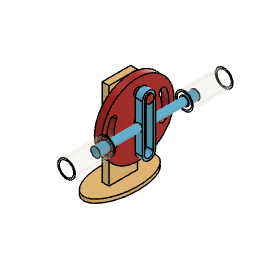
Scotch Yoke Mechanism v7 (Autodesk Fusion 360 design; units mm, degrees)
Autodesk Fusion 360 part; units mm, degrees
sketch "crank and pin" plane through (0, 0, 0) normal (1, 0, 0) x (0, 1, 0) in component "crank"
  circle A0 centre (0, 0) radius 50
  circle A1 centre (0, 33) radius 6
  line L0 (-50, 0) -> (50, 0) construction
  line L1 (0, 50) -> (0, -50) construction
  arc A2 (-30.2565, 13.1735) -> (-39.3225, 17.3995) centre (-34.4333, 16.0506) ccw
  arc A3 (-39.3225, -17.3995) -> (-30.2565, -13.1735) centre (-34.4333, -16.0506) ccw
  arc A4 (-38.6101, 18.9278) -> (-38.6101, -18.9278) centre (0, 0) ccw
  arc A5 (-29.5442, 14.7018) -> (-29.5442, -14.7018) centre (0, 0) ccw
  arc A6 (29.5442, -14.7018) -> (29.5442, 14.7018) centre (0, 0) ccw
  arc A7 (38.6101, -18.9278) -> (38.6101, 18.9278) centre (0, 0) ccw
  arc A8 (39.3225, 17.3995) -> (30.2565, 13.1735) centre (34.4333, 16.0506) ccw
  arc A9 (30.2565, -13.1735) -> (39.3225, -17.3995) centre (34.4333, -16.0506) ccw
  circle A10 centre (0, 0) radius 5
  dimension "d1" = 100
  dimension "d2" = 12
  dimension "d27" = 10
  constraint coincident A0.centre A4.centre
  constraint coincident A0 L0.start
  constraint coincident A0 L0.end
  constraint horizontal L0
  constraint coincident A0 L1.start
  constraint coincident A0 L1.end
  constraint vertical L1
  constraint symmetric L0 A2 A3
  constraint coincident A3 A4.end
  constraint coincident A3 A5.end
  constraint coincident A2 A4.start
  constraint coincident A2 A5.start
  constraint symmetric L1 A2.end A8.start
  constraint symmetric L1 A2.start A8.end
  constraint symmetric L1 A2 A8
  constraint symmetric L1 A3.end A9.start
  constraint symmetric L1 A3.start A9.end
  constraint symmetric L1 A3 A9
  constraint symmetric L1 A4.end A7.start
  constraint symmetric L1 A5.end A6.start
  constraint symmetric L1 A4.start A7.end
  constraint symmetric L1 A4 A7
  constraint symmetric L1 A5.start A6.end
  constraint symmetric L1 A5 A6
  constraint concentric A0 A10
  measures "d1" diameter of A0
  measures "d2" diameter of A1
  measures "d27" diameter of A10
extrude "Extrude1" add sketch "crank and pin" along normal blind 10 contours A0 | A1 | A2 A5 | A2 A3 A4 A5 | A3 A5 | A2 A4 | A3 A4 | A6 A9 | A6 A7 A8 A9 | A7 A9 | A6 A8 | A7 A8 | A10 makes body 1 in component "crank"
extrude "Extrude2" add sketch "crank and pin" along normal blind 20 contours A1 bodies 1 in component "crank"
extrude "Extrude3" cut sketch "crank and pin" along normal blind 40 contours A2 A3 A4 A5 bodies 1 in component "crank"
extrude "Extrude4" cut sketch "crank and pin" along normal blind 10 contours A6 A7 A8 A9 bodies 1 in component "crank"
ref_plane "WorkPlane1" through (15, 0, 0) normal (1, 0, 0) x (0, 1, 0) in component "sliding yoke"
sketch "sliding yoke main" plane through (15, 0, 0) normal (1, 0, 0) x (0, 1, 0) in component "sliding yoke"
  circle A0 centre (0, 33) radius 9
  line L0 (-50, 0) -> (50, 0) construction
  circle A1 centre (0, -33) radius 9
  circle A2 centre (0, 33) radius 6
  circle A3 centre (0, -33) radius 6
  line L1 (9, -33) -> (9, 33)
  line L2 (-9, 33) -> (-9, -33)
  line L3 (6, -33) -> (6, 33)
  line L4 (-6, 33) -> (-6, -33)
  dimension "d14" = 18
  dimension "d15" = 12
  constraint horizontal L0
  constraint symmetric A0 L0 A1
  constraint concentric A0 A2
  constraint symmetric L0 A2 A3
  constraint coincident A1 L1.start
  constraint coincident A0 L1.end
  constraint tangent A0 L1
  constraint perpendicular L0 L1
  constraint coincident A0 L2.start
  constraint coincident A1 L2.end
  constraint tangent A1 L2
  constraint parallel L1 L2
  constraint coincident A3 L3.start
  constraint coincident A2 L3.end
  constraint tangent A2 L3
  constraint parallel L1 L3
  constraint coincident A2 L4.start
  constraint coincident A3 L4.end
  constraint tangent A3 L4
  constraint perpendicular L0 L4
  measures "d14" diameter of A0
  measures "d15" diameter of A2
extrude "Extrude1'" add sketch "sliding yoke main" along normal blind 10 separate body contours A0 A2 L3 L4 | A0 A1 L1 L3 | A0 A1 L2 L4 | A1 A3 L3 L4 picked at (7.7444, 34.9209) picked at (7.9665, -33.4471) makes body 2 in component "sliding yoke"
extrude "Extrude5" add 1 faces at (20, 1.0163, 31.0501) along direction (1, 0, 0) blind 7 on bodies 1 bodies 1 in component "crank"
move_face "OffsetFaces1" offset -0.3 1 faces at (15.6667, 5.9702, 33.5974) on bodies 1 in component "crank"
sketch "sliding yoke left" plane through (0, -9, 0) normal (0, -1, 0) x (1, 0, 0) in component "sliding yoke"
  line L0 (15, 33) -> (15, -33)
  line L1 (15, -33) -> (25, -33)
  line L2 (25, -33) -> (25, 33)
  line L3 (25, 33) -> (15, 33)
  circle A0 centre (20, 0) radius 5
  dimension "d21" = 10
  measures "d21" diameter of A0
sketch "sliding yoke right" plane through (0, 9, 0) normal (0, 1, 0) x (-1, 0, 0) in component "sliding yoke"
  line L0 (-15, -33) -> (-15, 33)
  line L1 (-15, 33) -> (-25, 33)
  line L2 (-25, 33) -> (-25, -33)
  line L3 (-25, -33) -> (-15, -33)
  circle A0 centre (-20, 0) radius 5
  dimension "d22" = 10
  measures "d22" diameter of A0
extrude "Extrude2'" add sketch "sliding yoke right" along normal blind 60 contours A0 bodies 2 in component "sliding yoke"
extrude "Extrude3'" add sketch "sliding yoke left" along normal blind 60 contours A0 bodies 2 in component "sliding yoke"
extrude "Extrude6" cut sketch "crank and pin" along normal blind 10 contours A10 bodies 1 in component "crank"
ref_plane "WorkPlane1" through (-10, 0, 0) normal (1, 0, 0) x (0, 1, 0) in component "crank holder"
sketch "holder" plane through (-10, 0, 0) normal (1, 0, 0) x (0, 1, 0) in component "crank holder"
  line L0 (20, 40) -> (-20, 40)
  line L1 (-20, 40) -> (-20, -80)
  line L2 (-20, -80) -> (20, -80)
  line L3 (20, -80) -> (20, 40)
  circle A0 centre (0, 0) radius 5
  constraint horizontal L0
  constraint vertical L1
  constraint horizontal L2
  constraint vertical L3
  constraint coincident A0.centre origin
extrude "Extrude1''" add sketch "holder" against normal blind 10 separate body makes body 3 in component "crank holder"
extrude "Extrude2''" add sketch "holder" along normal blind 22 and the other way blind 10 contours A0 bodies 3 in component "crank holder"
move_face "OffsetFaces1'" offset -0.3 1 faces at (4.6667, 4.9938, -0.2492) on bodies 3 in component "crank holder"
sketch "holder stand" plane through (0, 0, -80) normal (0, 0, -1) x (1, 0, 0) in component "holder stand"
  line L0 (-10, -20) -> (-10, 20)
  line L1 (-10, 20) -> (-20, 20)
  line L2 (-20, 20) -> (-20, -20)
  line L3 (-20, -20) -> (-10, -20)
  ellipse E0 centre (-15, 0) end of major axis (-15, -50) minor radius 25
  line L4 (-15, 50) -> (-15, -50)
  line L5 (-40, 0) -> (10, 0)
  dimension "d38" = 50
  constraint parallel L0 L4
  constraint coincident E0 L4.start
  constraint coincident E0 L4.end
  constraint coincident E0 L5.start
  constraint coincident E0 L5.end
  measures "d38" distance of E0
extrude "Extrude1'''" add sketch "holder stand" along normal blind 5 separate body contours L0 L3 E0 L4 L5 | L0 L1 E0 L4 L5 | L2 L3 E0 L4 L5 | L1 L2 E0 L4 L5 makes body 4 in component "holder stand"
extrude "Extrude3''" add 1 faces at (-13.3333, -6.6667, -80) along direction (0, 0, -1) blind 5 on bodies 3 bodies 3 in component "crank holder"
move_face "OffsetFaces2" offset -0.3 4 faces at (-10, 0.1171, -58.229) (-16.6667, 20, -43.3333) (-20, -6.6667, -1.6667) (-16.6667, -20, -1.6667) on bodies 3 in component "crank holder"
move_body "Move1" bodies 2 to x (1, 0, 0) y (0, 1, 0) z (0, 0, 1) at (0, 0, 85) in component "sliding yoke"
move_body "Move1'" bodies 1 to x (1, 0, 0) y (0, 1, 0) z (0, 0, 1) at (0, 0, 85) in component "crank"
move_body "Move1''" bodies 4 to x (1, 0, 0) y (0, 1, 0) z (0, 0, 1) at (0, 0, 85) in component "holder stand"
move_body "Move1'''" bodies 3 to x (1, 0, 0) y (0, 1, 0) z (0, 0, 1) at (0, 0, 85) in component "crank holder"
sketch "right detail" plane through (0, 69, 0) normal (0, 1, 0) x (-1, 0, 0) in component "sliding yoke"
  circle A0 centre (-20, 85) radius 5
  circle A1 centre (-20, 85) radius 6.5
  dimension "d52" = 13
  constraint concentric A0 A1
  measures "d52" diameter of A1
extrude "Extrude4'" add sketch "right detail" against normal blind 15 bodies 2 in component "sliding yoke"
sketch "left detail" plane through (0, -69, 0) normal (0, -1, 0) x (1, 0, 0) in component "sliding yoke"
  circle A0 centre (20, 85) radius 5
  circle A1 centre (20, 85) radius 6.5
  dimension "d55" = 13
  constraint concentric A0 A1
  measures "d55" diameter of A1
extrude "Extrude5'" add sketch "left detail" against normal blind 15 bodies 2 in component "sliding yoke"
ref_plane "WorkPlane1" through (20, -148.7, 85) normal (0, -1, 0) x (1, 0, 0) in component "pistons"
sketch "left piston" plane through (20, -148.7, 85) normal (0, -1, 0) x (1, 0, 0) in component "pistons"
  circle A0 centre (0, 0) radius 10
  circle A1 centre (0, 0) radius 12
  dimension "d59" = 20
  dimension "d60" = 24
  constraint coincident A0.centre A1.centre
  measures "d59" diameter of A0
  measures "d60" diameter of A1
extrude "Extrude1''''" add sketch "left piston" along normal blind -95 and the other way blind 40 separate body makes body 5 in component "pistons"
move_face "MoveFace1" to x (1, 0, 0) y (0, 1, 0) z (0, 0, 1) at (0, 35, 0) 1 faces at (31.9404, -90.3667, 83.8052) on bodies 5 in component "pistons"
sketch "right piston" plane through (0, 69.3, 0) normal (0, 1, 0) x (-1, 0, 0) in component "pistons"
  circle A0 centre (-20, 85) radius 6.5
  circle A1 centre (-20, 85) radius 10
  circle A2 centre (-20, 85) radius 12
  dimension "d65" = 20
  dimension "d66" = 24
  constraint concentric A0 A1
  constraint concentric A1 A2
  measures "d65" diameter of A1
  measures "d66" diameter of A2
extrude "Extrude2'''" add sketch "right piston" along normal blind 40 and the other way blind 15 separate body contours A2 makes body 6 in component "pistons"
component "crank" placed x (1, 0, 0) y (0, 1, 0) z (0, 0, 1) at (0, 0, 0)
component "sliding yoke" placed x (1, 0, 0) y (0, 1, 0) z (0, 0, 1) at (0, 0.3, 0)
component "crank holder" placed x (1, 0, 0) y (0, 1, 0) z (0, 0, 1) at (0, 0, 0)
component "holder stand" placed x (1, 0, 0) y (0, 1, 0) z (0, 0, 1) at (0, 0, 0)
component "pistons" placed x (1, 0, 0) y (0, 1, 0) z (0, 0, 1) at (0, 0, 0)
named bodies: "crank and pin", "sliding yoke", "crank holder", "holder stand", "left piston", "right piston"
